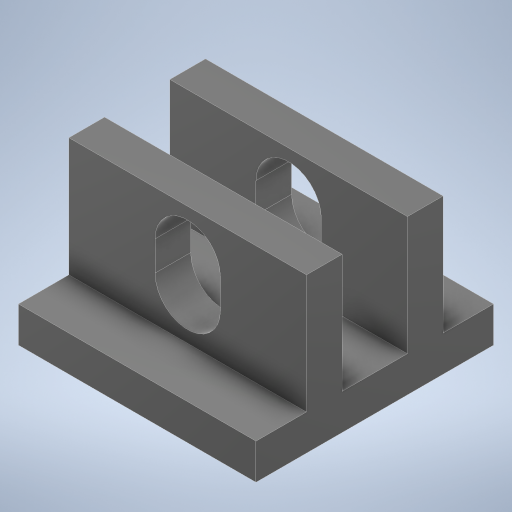
# Autodesk Inventor part: LegStablizer
Saved by Autodesk Inventor 2023 (Build 270158000, 158)
## iProperties
Created: 2023-11-27
Part Number: LegStablizer
Material: Thermoplastic Resin
Document SubType Name: Modeling
Designer: Mustapha
Mass: 2.78394 g
Surface Area: 19.4364 cm^2
Volume: 2.17495 cm^3
Density: 1.28 g/cm^3
Appearance: Smooth - Black
Author: Mustapha
Autodesk Inventor part; units mm, degrees
ref_plane "YZ Plane" through (0, 0, 0) normal (1, 0, 0) x (0, 1, 0)
ref_plane "XZ Plane" through (0, 0, 0) normal (0, 1, 0) x (-1, 0, 0)
ref_plane "XY Plane" through (0, 0, 0) normal (0, 0, 1) x (1, 0, 0)
sketch "Sketch1" plane through (0, 0, 0) normal (0, 1, 0) x (-1, 0, 0)
  line L0 (0, 0) -> (20, 0)
  line L1 (20, 0) -> (20, -20)
  line L2 (20, -20) -> (0, -20)
  line L3 (0, -20) -> (0, 0)
  dimension "d0" = 20
  dimension "d1" = 20
  constraints: 8 end point, 2 parallel, 1 horizontal, 1 perpendicular
  measures "d0" distance between parallel lines of L3 L1
  measures "d1" distance between parallel lines of L2 L0
extrude "Extrusion1" add sketch "Sketch1" along normal blind 3
sketch "Sketch2" plane through (0, 3, 0) normal (0, 1, 0) x (1, 0, 0)
  line L0 (-20, 20) -> (-20, 0) projected
  line L1 (0, 0) -> (0, 20) projected
  line L2 (-20, 4.25) -> (0, 4.25)
  line L3 (0, 4.25) -> (0, 7.25)
  line L4 (0, 7.25) -> (-20, 7.25)
  line L5 (-20, 7.25) -> (-20, 4.25)
  line L6 (-20, 15.75) -> (0, 15.75)
  line L7 (0, 15.75) -> (0, 12.75)
  line L8 (0, 12.75) -> (-20, 12.75)
  line L9 (-20, 12.75) -> (-20, 15.75)
  line L10 (0, 20) -> (-20, 20) projected
  point P0 (0, 15.75)
  point P1 (0, 4.25)
  dimension "d4" = 3
  dimension "d5" = 3
  dimension "d6" = 5.5
  dimension "d7" = 4.25
  constraints: 16 end point, 4 parallel, 4 point on line, 2 horizontal, 2 perpendicular
  measures "d4" distance between parallel lines of L4 L2
  measures "d5" distance between parallel lines of L6 L8
  measures "d6" distance between parallel lines of L8 L4
  measures "d7" distance between parallel lines of L10 L6
extrude "Extrusion2" add sketch "Sketch2" along normal blind 10 contours L6 L1 L8 L0 | L4 L1 L2 L0
sketch "Sketch3" plane through (-20, 3, -4.25) normal (0, 0, 1) x (1, 0, 0)
  line L0 (10, 6.25) -> (10, 3.75) construction
  line L1 (0, 10) -> (20, 10) projected
  line L2 (7.25, 6.25) -> (7.25, 3.75)
  line L3 (12.75, 3.75) -> (12.75, 6.25)
  arc A0 (12.75, 6.25) -> (7.25, 6.25) centre (10, 6.25) ccw
  arc A1 (7.25, 3.75) -> (12.75, 3.75) centre (10, 3.75) ccw
  line L4 (0, 0) -> (0, 10) projected
  point P0 (20, -3)
  point P1 (10, 5)
  point P2 (10, 1)
  point P3 (10, 9)
  dimension "d10" = 5.5
  dimension "d11" = 10
  dimension "d12" = 8
  dimension "d13" = 9
  constraints: 8 end point, 6 point on circle, 4 tangent, 2 centre point, 1 midpoint, 1 parallel, 1 perpendicular
  measures "d10" distance between parallel lines of L3 L2
  measures "d11" distance between parallel lines of L4 L0
  measures "d12" distance of point (10, 1) point (10, 9)
extrude "Extrusion3" cut sketch "Sketch3" against normal blind 16.75
body "Solid1"
